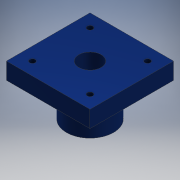
# Autodesk Inventor part: soporte
Saved by Autodesk Inventor 2018 (Build 220112000, 112)
## iProperties
Created: 2018-01-01
Part Number: soporte
Material: Genérico
Document SubType Name: Modeling
Designer: Carlos
Density: 1 g/cm^3
Appearance: Valor por defecto
Author: Carlos
Autodesk Inventor part; units mm, degrees
ref_plane "YZ Plane" through (0, 0, 0) normal (1, 0, 0) x (0, 1, 0)
ref_plane "XZ Plane" through (0, 0, 0) normal (0, 1, 0) x (-1, 0, 0)
ref_plane "XY Plane" through (0, 0, 0) normal (0, 0, 1) x (1, 0, 0)
sketch "Boceto1" plane through (0, 0, 0) normal (0, 0, 1) x (1, 0, 0)
  line L0 (-22.5, -22.5) -> (22.5, -22.5)
  line L1 (22.5, -22.5) -> (22.5, 22.5)
  line L2 (22.5, 22.5) -> (-22.5, 22.5)
  line L3 (-22.5, 22.5) -> (-22.5, -22.5)
  line L4 (-22.5, -22.5) -> (22.5, 22.5) construction
  line L5 (22.5, -22.5) -> (-22.5, 22.5) construction
  point P0 (0, 0)
  dimension "d0" = 45
  dimension "d1" = 45
  constraints: 12 end point, 2 midpoint, 2 parallel, 1 horizontal, 1 perpendicular
  measures "d0" distance of L1.end L2.end
  measures "d1" distance of L0.end L1.end
extrude "Extrusión1" add sketch "Boceto1" along normal blind 9
sketch "Boceto2" plane through (0, 0, 9) normal (0, 0, 1) x (1, 0, 0)
  circle A0 centre (0, 0) radius 6
  dimension "d4" = 12
  constraints: 1 centre point, 1 coincident
  measures "d4" diameter of A0
hole "Agujero1" at (0, 0, 9) direction (0, 0, -1) diameter 12 depth 9
sketch "Boceto3" plane through (0, 0, 9) normal (0, 0, 1) x (1, 0, 0)
  line L0 (-15.5, -15.5) -> (15.5, -15.5)
  line L1 (15.5, -15.5) -> (15.5, 15.5)
  line L2 (15.5, 15.5) -> (-15.5, 15.5)
  line L3 (-15.5, 15.5) -> (-15.5, -15.5)
  line L4 (-15.5, -15.5) -> (15.5, 15.5) construction
  line L5 (15.5, -15.5) -> (-15.5, 15.5) construction
  line L6 (0, 15.5) -> (0, -15.5)
  line L7 (-15.5, 0) -> (15.5, 0)
  point P0 (0, 0)
  dimension "d12" = 31
  dimension "d13" = 31
  constraints: 16 end point, 6 midpoint, 2 parallel, 1 horizontal, 1 perpendicular
  measures "d12" distance of L1.end L2.end
  measures "d13" distance of L0.end L1.end
hole "Agujero2" at (-15.5, 15.5, 9) at (-15.5, -15.5, 9) at (15.5, -15.5, 9) at (15.5, 15.5, 9) direction (0, 0, -1) diameter 3 depth 9 tip angle 118
sketch "Boceto4" plane through (0, 0, 0) normal (0, 0, -1) x (-1, 0, 0)
  circle A0 centre (0, 0) radius 12.7
  dimension "d21" = 25.4
  constraints: 1 centre point, 1 coincident
  measures "d21" diameter of A0
extrude "Extrusión2" add sketch "Boceto4" along normal blind 18
